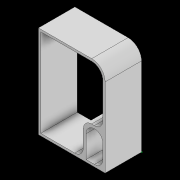
# Autodesk Inventor part: ElecTweetBox
Saved by Autodesk Inventor 2022 (Build 260153000, 153)
## iProperties
Created: 2022-07-12
Part Number: ElecTweetBox
Material: Generic
Document SubType Name: Modeling
Designer: Fuzzyfish
Density: 1 g/cm^3
Appearance: Default
Author: Fuzzyfish
Autodesk Inventor part; units mm, degrees
ref_plane "YZ Plane" through (0, 0, 0) normal (1, 0, 0) x (0, 1, 0)
ref_plane "XZ Plane" through (0, 0, 0) normal (0, 1, 0) x (-1, 0, 0)
ref_plane "XY Plane" through (0, 0, 0) normal (0, 0, 1) x (1, 0, 0)
sketch "Sketch1" plane through (0, 0, 0) normal (0, 0, 1) x (1, 0, 0)
  line L0 (0, 0) -> (119, 0)
  line L1 (119, 0) -> (119, 141)
  arc A0 (119, 141) -> (95, 165) centre (95, 141) ccw
  line L2 (0, 0) -> (0, 165)
  line L3 (0, 165) -> (95, 165)
  dimension "d0" = 24
  dimension "d1" = 95
  dimension "d2" = 165
  constraints: 8 end point, 2 horizontal, 2 point on circle, 2 tangent, 1 centre point, 1 perpendicular, 1 vertical
  measures "d0" radius of A0
  measures "d1" distance of L2.end L3.end
  measures "d2" distance of L0.start L2.end
extrude "Extrusion1" add sketch "Sketch1" along normal blind 65
shell "Shell1" thickness 4 removed faces 2 at (39.6667, 102, 65) at (39.6667, 102, 0)
fillet "Fillet1" radius 15 1 edges at (115, 4, 32.5)
sketch "Sketch3" plane through (0, 0, 0) normal (0, 0, -1) x (-1, 0, 0)
  line L0 (-115, 19) -> (-115, 141) projected
  line L1 (0, 0) -> (-119, 0) projected
  line L2 (-119, 0) -> (-85, 0)
  line L3 (-85, 0) -> (-85, 59)
  line L4 (-85, 59) -> (-119, 59)
  line L5 (-119, 59) -> (-119, 0)
  line L6 (-119, 0) -> (-80, 0)
  line L7 (-80, 0) -> (-80, 64)
  line L8 (-80, 64) -> (-119, 64)
  line L9 (-119, 64) -> (-119, 0)
  line L10 (-4, 4) -> (-100, 4) projected
  point P0 (-85, 4)
  point P1 (-80, 4)
  point P2 (-115, 64)
  point P3 (-115, 59)
  dimension "d22" = 5
  dimension "d23" = 5
  dimension "d24" = 30
  dimension "d25" = 55
  constraints: 16 end point, 4 parallel, 2 horizontal, 2 perpendicular
  measures "d22" distance between parallel lines of L3 L7
  measures "d23" distance between parallel lines of L8 L4
  measures "d24" distance between parallel lines of L0 L3
  measures "d25" distance between parallel lines of L10 L4
extrude "Extrusion4" add sketch "Sketch3" against normal blind 65 contours L0 L8 L7 L10 L3 L4
fillet "Fillet3" radius 15 5 edges at (80, 64, 32.5) (115, 64, 32.5) (80, 4, 32.5) (85, 59, 32.5) (115, 59, 32.5)
sketch "Sketch4" plane through (119, 0, 0) normal (1, 0, 0) x (0, 0, -1)
  point P0 (0, 0)
body "Solid1"
